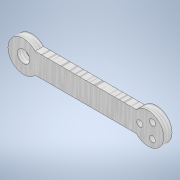
# Autodesk Inventor part: 駆動軸抑え
Saved by Autodesk Inventor 2020.2 (Build 242310000, 310)
## iProperties
Created: 2020-03-15
Part Number: 駆動軸抑え
Material: アルミニウム 7075
Document SubType Name: Modeling
Designer: aoyam
Density: 2.81 g/cm^3
Appearance: サテン - ブラシ仕上げ 重厚
Author: aoyam
Autodesk Inventor part; units mm, degrees
ref_plane "YZ Plane" through (0, 0, 0) normal (1, 0, 0) x (0, 1, 0)
ref_plane "XZ Plane" through (0, 0, 0) normal (0, 1, 0) x (-1, 0, 0)
ref_plane "XY Plane" through (0, 0, 0) normal (0, 0, 1) x (1, 0, 0)
sketch "スケッチ1" plane through (0, 0, 0) normal (0, 0, 1) x (1, 0, 0)
  arc A0 (2.3922, 20.2558) -> (2.3331, 19.9425) centre (4.2654, 19.7401) ccw
  arc A1 (2.759, 21.2362) -> (2.3922, 20.2558) centre (7.5685, 18.8782) ccw
  arc A2 (3.8916, 23.0137) -> (2.759, 21.2362) centre (11.1286, 17.1527) ccw
  arc A3 (-0.0572, 19.9425) -> (-0.1163, 20.2558) centre (-1.9895, 19.7401) ccw
  arc A4 (-0.1163, 20.2558) -> (-0.4831, 21.2362) centre (-5.2926, 18.8782) ccw
  arc A5 (-0.4831, 21.2362) -> (-1.6157, 23.0137) centre (-8.8527, 17.1527) ccw
  arc A6 (2.2508, 18.6513) -> (0.0251, 18.6513) centre (1.1379, 1.1867) ccw
  arc A7 (-1.6157, 23.0137) -> (-2.9881, 22.7963) centre (1.1379, 1.1867) ccw
  line L0 (2.2508, 18.6513) -> (2.3331, 19.9425)
  line L1 (0.0251, 18.6513) -> (-0.0572, 19.9425)
  line L2 (-5.3173, 17.4526) -> (-5.7946, 18.6552)
  arc A8 (-5.7946, 18.6552) -> (-5.9476, 18.9349) centre (-7.5698, 17.8656) ccw
  arc A9 (-5.9476, 18.9349) -> (-6.5994, 19.754) centre (-10.4448, 16.0252) ccw
  arc A10 (-6.5994, 19.754) -> (-8.2258, 21.0945) centre (-13.2975, 13.284) ccw
  arc A11 (-8.2258, 21.0945) -> (-9.4639, 20.4637) centre (1.1379, 1.1867) ccw
  arc A12 (-3.2005, 18.1404) -> (-5.3173, 17.4526) centre (1.1379, 1.1867) ccw
  line L3 (-3.2005, 18.1404) -> (-3.5213, 19.3939)
  arc A13 (-3.5619, 19.71) -> (-3.5213, 19.3939) centre (-1.621, 19.7985) ccw
  arc A14 (-3.516, 20.7559) -> (-3.5619, 19.71) centre (1.7868, 19.9995) ccw
  arc A15 (-2.9881, 22.7963) -> (-3.516, 20.7559) centre (5.7058, 19.4586) ccw
  line L4 (-10.0278, 14.6617) -> (-10.8533, 15.658)
  arc A16 (-10.8533, 15.658) -> (-11.0853, 15.8767) centre (-12.2977, 14.3585) ccw
  arc A17 (-11.0853, 15.8767) -> (-11.9583, 16.4543) centre (-14.4633, 11.7197) ccw
  arc A18 (-11.9583, 16.4543) -> (-13.9194, 17.2266) centre (-16.3293, 8.2311) ccw
  arc A19 (-13.9194, 17.2266) -> (-14.9019, 16.244) centre (1.1379, 1.1867) ccw
  arc A20 (-8.2272, 15.97) -> (-10.0278, 14.6617) centre (1.1379, 1.1867) ccw
  line L5 (-8.2272, 15.97) -> (-8.9196, 17.063)
  arc A21 (-9.0559, 17.3511) -> (-8.9196, 17.063) centre (-7.2373, 18.035) ccw
  arc A22 (-9.3354, 18.3599) -> (-9.0559, 17.3511) centre (-4.0584, 19.2792) ccw
  arc A23 (-9.4639, 20.4637) -> (-9.3354, 18.3599) centre (-0.164, 19.9759) ccw
  line L6 (-13.6453, 10.5518) -> (-14.7383, 11.2442)
  arc A24 (-14.7383, 11.2442) -> (-15.0265, 11.3805) centre (-15.7104, 9.562) ccw
  arc A25 (-15.0265, 11.3805) -> (-16.0353, 11.6601) centre (-16.9545, 6.3831) ccw
  arc A26 (-16.0353, 11.6601) -> (-18.139, 11.7886) centre (-17.6512, 2.4887) ccw
  arc A27 (-18.139, 11.7886) -> (-18.7698, 10.5505) centre (1.1379, 1.1867) ccw
  arc A28 (-12.3371, 12.3525) -> (-13.6453, 10.5518) centre (1.1379, 1.1867) ccw
  line L7 (-12.3371, 12.3525) -> (-13.3333, 13.178)
  arc A29 (-13.552, 13.4099) -> (-13.3333, 13.178) centre (-12.0338, 14.6223) ccw
  arc A30 (-14.1296, 14.283) -> (-13.552, 13.4099) centre (-9.395, 16.7879) ccw
  arc A31 (-14.9019, 16.244) -> (-14.1296, 14.283) centre (-5.9065, 18.6539) ccw
  line L8 (-15.8158, 5.5252) -> (-17.0692, 5.8459)
  arc A32 (-17.0692, 5.8459) -> (-17.3854, 5.8865) centre (-17.4739, 3.9456) ccw
  arc A33 (-17.3854, 5.8865) -> (-18.4312, 5.8407) centre (-17.6748, 0.5379) ccw
  arc A34 (-18.4312, 5.8407) -> (-20.4717, 5.3128) centre (-17.1339, -3.3812) ccw
  arc A35 (-20.4717, 5.3128) -> (-20.6891, 3.9404) centre (1.1379, 1.1867) ccw
  arc A36 (-15.128, 7.642) -> (-15.8158, 5.5252) centre (1.1379, 1.1867) ccw
  line L9 (-15.128, 7.642) -> (-16.3306, 8.1192)
  arc A37 (-16.6102, 8.2722) -> (-16.3306, 8.1192) centre (-15.541, 9.8944) ccw
  arc A38 (-17.4293, 8.924) -> (-16.6102, 8.2722) centre (-13.7005, 12.7695) ccw
  arc A39 (-18.7698, 10.5505) -> (-17.4293, 8.924) centre (-10.9594, 15.6222) ccw
  line L10 (-16.3266, 0.0739) -> (-17.6179, -0.0084)
  arc A40 (-17.6179, -0.0084) -> (-17.9311, -0.0675) centre (-17.4155, -1.9407) ccw
  arc A41 (-17.9311, -0.0675) -> (-18.9116, -0.4343) centre (-16.5535, -5.2438) ccw
  arc A42 (-18.9116, -0.4343) -> (-20.6891, -1.5669) centre (-14.8281, -8.8039) ccw
  arc A43 (-20.6891, -1.5669) -> (-20.4717, -2.9393) centre (1.1379, 1.1867) ccw
  arc A44 (-16.3266, 2.2996) -> (-16.3266, 0.0739) centre (1.1379, 1.1867) ccw
  line L11 (-16.3266, 2.2996) -> (-17.6179, 2.3819)
  arc A45 (-17.9311, 2.441) -> (-17.6179, 2.3819) centre (-17.4155, 4.3142) ccw
  arc A46 (-18.9116, 2.8078) -> (-17.9311, 2.441) centre (-16.5535, 7.6173) ccw
  arc A47 (-20.6891, 3.9404) -> (-18.9116, 2.8078) centre (-14.8281, 11.1774) ccw
  line L12 (-15.128, -5.2685) -> (-16.3306, -5.7458)
  arc A48 (-16.3306, -5.7458) -> (-16.6102, -5.8988) centre (-15.541, -7.521) ccw
  arc A49 (-16.6102, -5.8988) -> (-17.4293, -6.5506) centre (-13.7005, -10.396) ccw
  arc A50 (-17.4293, -6.5506) -> (-18.7698, -8.177) centre (-10.9594, -13.2487) ccw
  arc A51 (-18.7698, -8.177) -> (-18.139, -9.4151) centre (1.1379, 1.1867) ccw
  arc A52 (-15.8158, -3.1517) -> (-15.128, -5.2685) centre (1.1379, 1.1867) ccw
  line L13 (-15.8158, -3.1517) -> (-17.0692, -3.4725)
  arc A53 (-17.3854, -3.5131) -> (-17.0692, -3.4725) centre (-17.4739, -1.5722) ccw
  arc A54 (-18.4312, -3.4672) -> (-17.3854, -3.5131) centre (-17.6748, 1.8356) ccw
  arc A55 (-20.4717, -2.9393) -> (-18.4312, -3.4672) centre (-17.1339, 5.7546) ccw
  line L14 (-12.3371, -9.979) -> (-13.3333, -10.8046)
  arc A56 (-13.3333, -10.8046) -> (-13.552, -11.0365) centre (-12.0338, -12.2489) ccw
  arc A57 (-13.552, -11.0365) -> (-14.1296, -11.9095) centre (-9.395, -14.4145) ccw
  arc A58 (-14.1296, -11.9095) -> (-14.9019, -13.8706) centre (-5.9065, -16.2805) ccw
  arc A59 (-14.9019, -13.8706) -> (-13.9194, -14.8531) centre (1.1379, 1.1867) ccw
  arc A60 (-13.6453, -8.1784) -> (-12.3371, -9.979) centre (1.1379, 1.1867) ccw
  line L15 (-13.6453, -8.1784) -> (-14.7383, -8.8708)
  arc A61 (-15.0265, -9.0071) -> (-14.7383, -8.8708) centre (-15.7104, -7.1885) ccw
  arc A62 (-16.0353, -9.2866) -> (-15.0265, -9.0071) centre (-16.9545, -4.0097) ccw
  arc A63 (-18.139, -9.4151) -> (-16.0353, -9.2866) centre (-17.6512, -0.1153) ccw
  line L16 (-8.2272, -13.5965) -> (-8.9196, -14.6895)
  arc A64 (-8.9196, -14.6895) -> (-9.0559, -14.9777) centre (-7.2373, -15.6616) ccw
  arc A65 (-9.0559, -14.9777) -> (-9.3354, -15.9865) centre (-4.0584, -16.9058) ccw
  arc A66 (-9.3354, -15.9865) -> (-9.4639, -18.0902) centre (-0.164, -17.6024) ccw
  arc A67 (-9.4639, -18.0902) -> (-8.2258, -18.7211) centre (1.1379, 1.1867) ccw
  arc A68 (-10.0278, -12.2883) -> (-8.2272, -13.5965) centre (1.1379, 1.1867) ccw
  line L17 (-10.0278, -12.2883) -> (-10.8533, -13.2846)
  arc A69 (-11.0853, -13.5032) -> (-10.8533, -13.2846) centre (-12.2977, -11.985) ccw
  arc A70 (-11.9583, -14.0808) -> (-11.0853, -13.5032) centre (-14.4633, -9.3462) ccw
  arc A71 (-13.9194, -14.8531) -> (-11.9583, -14.0808) centre (-16.3293, -5.8577) ccw
  line L18 (-3.2005, -15.767) -> (-3.5213, -17.0204)
  arc A72 (-3.5213, -17.0204) -> (-3.5619, -17.3366) centre (-1.621, -17.4251) ccw
  arc A73 (-3.5619, -17.3366) -> (-3.516, -18.3824) centre (1.7868, -17.626) ccw
  arc A74 (-3.516, -18.3824) -> (-2.9881, -20.4229) centre (5.7058, -17.0851) ccw
  arc A75 (-2.9881, -20.4229) -> (-1.6157, -20.6403) centre (1.1379, 1.1867) ccw
  arc A76 (-5.3173, -15.0792) -> (-3.2005, -15.767) centre (1.1379, 1.1867) ccw
  line L19 (-5.3173, -15.0792) -> (-5.7946, -16.2818)
  arc A77 (-5.9476, -16.5614) -> (-5.7946, -16.2818) centre (-7.5698, -15.4922) ccw
  arc A78 (-6.5994, -17.3806) -> (-5.9476, -16.5614) centre (-10.4448, -13.6517) ccw
  arc A79 (-8.2258, -18.7211) -> (-6.5994, -17.3806) centre (-13.2975, -10.9106) ccw
  line L20 (2.2508, -16.2779) -> (2.3331, -17.5691)
  arc A80 (2.3331, -17.5691) -> (2.3922, -17.8823) centre (4.2654, -17.3667) ccw
  arc A81 (2.3922, -17.8823) -> (2.759, -18.8628) centre (7.5685, -16.5048) ccw
  arc A82 (2.759, -18.8628) -> (3.8916, -20.6403) centre (11.1286, -14.7793) ccw
  arc A83 (3.8916, -20.6403) -> (5.264, -20.4229) centre (1.1379, 1.1867) ccw
  arc A84 (0.0251, -16.2779) -> (2.2508, -16.2779) centre (1.1379, 1.1867) ccw
  line L21 (0.0251, -16.2779) -> (-0.0572, -17.5691)
  arc A85 (-0.1163, -17.8823) -> (-0.0572, -17.5691) centre (-1.9895, -17.3667) ccw
  arc A86 (-0.4831, -18.8628) -> (-0.1163, -17.8823) centre (-5.2926, -16.5048) ccw
  arc A87 (-1.6157, -20.6403) -> (-0.4831, -18.8628) centre (-8.8527, -14.7793) ccw
  line L22 (7.5932, -15.0792) -> (8.0705, -16.2818)
  arc A88 (8.0705, -16.2818) -> (8.2235, -16.5614) centre (9.8457, -15.4922) ccw
  arc A89 (8.2235, -16.5614) -> (8.8753, -17.3806) centre (12.7207, -13.6517) ccw
  arc A90 (8.8753, -17.3806) -> (10.5017, -18.7211) centre (15.5734, -10.9106) ccw
  arc A91 (10.5017, -18.7211) -> (11.7398, -18.0902) centre (1.1379, 1.1867) ccw
  arc A92 (5.4764, -15.767) -> (7.5932, -15.0792) centre (1.1379, 1.1867) ccw
  line L23 (5.4764, -15.767) -> (5.7971, -17.0204)
  arc A93 (5.8377, -17.3366) -> (5.7971, -17.0204) centre (3.8969, -17.4251) ccw
  arc A94 (5.7919, -18.3824) -> (5.8377, -17.3366) centre (0.4891, -17.626) ccw
  arc A95 (5.264, -20.4229) -> (5.7919, -18.3824) centre (-3.43, -17.0851) ccw
  line L24 (12.3037, -12.2883) -> (13.1292, -13.2846)
  arc A96 (13.1292, -13.2846) -> (13.3611, -13.5032) centre (14.5735, -11.985) ccw
  arc A97 (13.3611, -13.5032) -> (14.2342, -14.0808) centre (16.7391, -9.3462) ccw
  arc A98 (14.2342, -14.0808) -> (16.1953, -14.8531) centre (18.6051, -5.8577) ccw
  arc A99 (16.1953, -14.8531) -> (17.1778, -13.8706) centre (1.1379, 1.1867) ccw
  arc A100 (10.503, -13.5965) -> (12.3037, -12.2883) centre (1.1379, 1.1867) ccw
  line L25 (10.503, -13.5965) -> (11.1954, -14.6895)
  arc A101 (11.3317, -14.9777) -> (11.1954, -14.6895) centre (9.5132, -15.6616) ccw
  arc A102 (11.6113, -15.9865) -> (11.3317, -14.9777) centre (6.3343, -16.9058) ccw
  arc A103 (11.7398, -18.0902) -> (11.6113, -15.9865) centre (2.4399, -17.6024) ccw
  line L26 (15.9212, -8.1784) -> (17.0142, -8.8708)
  arc A104 (17.0142, -8.8708) -> (17.3023, -9.0071) centre (17.9862, -7.1885) ccw
  arc A105 (17.3023, -9.0071) -> (18.3111, -9.2866) centre (19.2304, -4.0097) ccw
  arc A106 (18.3111, -9.2866) -> (20.4149, -9.4151) centre (19.9271, -0.1153) ccw
  arc A107 (20.4149, -9.4151) -> (21.0457, -8.177) centre (1.1379, 1.1867) ccw
  arc A108 (14.6129, -9.979) -> (15.9212, -8.1784) centre (1.1379, 1.1867) ccw
  line L27 (14.6129, -9.979) -> (15.6092, -10.8046)
  arc A109 (15.8279, -11.0365) -> (15.6092, -10.8046) centre (14.3097, -12.2489) ccw
  arc A110 (16.4055, -11.9095) -> (15.8279, -11.0365) centre (11.6709, -14.4145) ccw
  arc A111 (17.1778, -13.8706) -> (16.4055, -11.9095) centre (8.1824, -16.2805) ccw
  line L28 (18.0916, -3.1517) -> (19.3451, -3.4725)
  arc A112 (19.3451, -3.4725) -> (19.6613, -3.5131) centre (19.7497, -1.5722) ccw
  arc A113 (19.6613, -3.5131) -> (20.7071, -3.4672) centre (19.9507, 1.8356) ccw
  arc A114 (20.7071, -3.4672) -> (22.7476, -2.9393) centre (19.4098, 5.7546) ccw
  arc A115 (22.7476, -2.9393) -> (22.9649, -1.5669) centre (1.1379, 1.1867) ccw
  arc A116 (17.4038, -5.2685) -> (18.0916, -3.1517) centre (1.1379, 1.1867) ccw
  line L29 (17.4038, -5.2685) -> (18.6065, -5.7458)
  arc A117 (18.8861, -5.8988) -> (18.6065, -5.7458) centre (17.8168, -7.521) ccw
  arc A118 (19.7052, -6.5506) -> (18.8861, -5.8988) centre (15.9764, -10.396) ccw
  arc A119 (21.0457, -8.177) -> (19.7052, -6.5506) centre (13.2352, -13.2487) ccw
  line L30 (18.6025, 2.2996) -> (19.8937, 2.3819)
  arc A120 (19.8937, 2.3819) -> (20.207, 2.441) centre (19.6914, 4.3142) ccw
  arc A121 (20.207, 2.441) -> (21.1874, 2.8078) centre (18.8294, 7.6173) ccw
  arc A122 (21.1874, 2.8078) -> (22.9649, 3.9404) centre (17.104, 11.1774) ccw
  arc A123 (22.9649, 3.9404) -> (22.7476, 5.3128) centre (1.1379, 1.1867) ccw
  arc A124 (18.6025, 0.0739) -> (18.6025, 2.2996) centre (1.1379, 1.1867) ccw
  line L31 (18.6025, 0.0739) -> (19.8937, -0.0084)
  arc A125 (20.207, -0.0675) -> (19.8937, -0.0084) centre (19.6914, -1.9407) ccw
  arc A126 (21.1874, -0.4343) -> (20.207, -0.0675) centre (18.8294, -5.2438) ccw
  arc A127 (22.9649, -1.5669) -> (21.1874, -0.4343) centre (17.104, -8.8039) ccw
  line L32 (17.4038, 7.642) -> (18.6065, 8.1192)
  arc A128 (18.6065, 8.1192) -> (18.8861, 8.2722) centre (17.8168, 9.8944) ccw
  arc A129 (18.8861, 8.2722) -> (19.7052, 8.924) centre (15.9764, 12.7695) ccw
  arc A130 (19.7052, 8.924) -> (21.0457, 10.5505) centre (13.2352, 15.6222) ccw
  arc A131 (21.0457, 10.5505) -> (20.4149, 11.7886) centre (1.1379, 1.1867) ccw
  arc A132 (18.0916, 5.5252) -> (17.4038, 7.642) centre (1.1379, 1.1867) ccw
  line L33 (18.0916, 5.5252) -> (19.3451, 5.8459)
  arc A133 (19.6613, 5.8865) -> (19.3451, 5.8459) centre (19.7497, 3.9456) ccw
  arc A134 (20.7071, 5.8407) -> (19.6613, 5.8865) centre (19.9507, 0.5379) ccw
  arc A135 (22.7476, 5.3128) -> (20.7071, 5.8407) centre (19.4098, -3.3812) ccw
  line L34 (14.6129, 12.3525) -> (15.6092, 13.178)
  arc A136 (15.6092, 13.178) -> (15.8279, 13.4099) centre (14.3097, 14.6223) ccw
  arc A137 (15.8279, 13.4099) -> (16.4055, 14.283) centre (11.6709, 16.7879) ccw
  arc A138 (16.4055, 14.283) -> (17.1778, 16.244) centre (8.1824, 18.6539) ccw
  arc A139 (17.1778, 16.244) -> (16.1953, 17.2266) centre (1.1379, 1.1867) ccw
  arc A140 (15.9212, 10.5518) -> (14.6129, 12.3525) centre (1.1379, 1.1867) ccw
  line L35 (15.9212, 10.5518) -> (17.0142, 11.2442)
  arc A141 (17.3023, 11.3805) -> (17.0142, 11.2442) centre (17.9862, 9.562) ccw
  arc A142 (18.3111, 11.6601) -> (17.3023, 11.3805) centre (19.2304, 6.3831) ccw
  arc A143 (20.4149, 11.7886) -> (18.3111, 11.6601) centre (19.9271, 2.4887) ccw
  line L36 (10.503, 15.97) -> (11.1954, 17.063)
  arc A144 (11.1954, 17.063) -> (11.3317, 17.3511) centre (9.5132, 18.035) ccw
  arc A145 (11.3317, 17.3511) -> (11.6113, 18.3599) centre (6.3343, 19.2792) ccw
  arc A146 (11.6113, 18.3599) -> (11.7398, 20.4637) centre (2.4399, 19.9759) ccw
  arc A147 (11.7398, 20.4637) -> (10.5017, 21.0945) centre (1.1379, 1.1867) ccw
  arc A148 (12.3037, 14.6617) -> (10.503, 15.97) centre (1.1379, 1.1867) ccw
  line L37 (12.3037, 14.6617) -> (13.1292, 15.658)
  arc A149 (13.3611, 15.8767) -> (13.1292, 15.658) centre (14.5735, 14.3585) ccw
  arc A150 (14.2342, 16.4543) -> (13.3611, 15.8767) centre (16.7391, 11.7197) ccw
  arc A151 (16.1953, 17.2266) -> (14.2342, 16.4543) centre (18.6051, 8.2311) ccw
  line L38 (5.4764, 18.1404) -> (5.7971, 19.3939)
  arc A152 (5.7971, 19.3939) -> (5.8377, 19.71) centre (3.8969, 19.7985) ccw
  arc A153 (5.8377, 19.71) -> (5.7919, 20.7559) centre (0.4891, 19.9995) ccw
  arc A154 (5.7919, 20.7559) -> (5.264, 22.7963) centre (-3.43, 19.4586) ccw
  arc A155 (5.264, 22.7963) -> (3.8916, 23.0137) centre (1.1379, 1.1867) ccw
  arc A156 (7.5932, 17.4526) -> (5.4764, 18.1404) centre (1.1379, 1.1867) ccw
  line L39 (7.5932, 17.4526) -> (8.0705, 18.6552)
  arc A157 (8.2235, 18.9349) -> (8.0705, 18.6552) centre (9.8457, 17.8656) ccw
  arc A158 (8.8753, 19.754) -> (8.2235, 18.9349) centre (12.7207, 16.0252) ccw
  arc A159 (10.5017, 21.0945) -> (8.8753, 19.754) centre (15.5734, 13.284) ccw
  circle A160 centre (1.1379, 1.1867) radius 3.025
  line L40 (1.1379, 1.1867) -> (61.1379, 1.1867)
  line L41 (66.1379, -3.8133) -> (-5.7946, -3.8133)
  line L42 (-5.7946, -3.8133) -> (-5.7946, 6.1867)
  line L43 (-5.7946, 6.1867) -> (66.1379, 6.1867)
  line L44 (66.1379, 6.1867) -> (66.1379, -3.8133)
  circle A161 centre (61.1379, 1.1867) radius 7.5
  circle A162 centre (1.1379, 1.1867) radius 7.5
  circle A163 centre (57.1379, 1.1867) radius 1.5
  circle A164 centre (63.1379, -2.2774) radius 1.5
  circle A165 centre (63.1379, 4.6508) radius 1.5
  line L45 (63.1379, -2.2774) -> (63.1379, 4.6508)
  point P0 (0, 0)
  point P1 (-10.0278, -12.2883)
  point P2 (-8.2272, -13.5965)
  point P3 (-8.9196, -14.6895)
  point P4 (-9.0559, -14.9777)
  point P5 (-9.3354, -15.9865)
  point P6 (-9.4639, -18.0902)
  point P7 (-8.2258, -18.7211)
  point P8 (-5.9476, -16.5614)
  point P9 (-5.7946, -16.2818)
  point P10 (-5.3173, -15.0792)
  point P11 (-3.2005, -15.767)
  point P12 (-3.5213, -17.0204)
  point P13 (-3.5619, -17.3366)
  point P14 (-3.516, -18.3824)
  point P15 (-2.9881, -20.4229)
  point P16 (-1.6157, -20.6403)
  point P17 (-0.4831, -18.8628)
  point P18 (-0.1163, -17.8823)
  point P19 (-0.0572, -17.5691)
  point P20 (0.0251, -16.2779)
  point P21 (2.2508, -16.2779)
  point P22 (2.3331, -17.5691)
  point P23 (2.3922, -17.8823)
  point P24 (2.759, -18.8628)
  point P25 (3.8916, -20.6403)
  point P26 (5.264, -20.4229)
  point P27 (5.7919, -18.3824)
  point P28 (5.8377, -17.3366)
  point P29 (5.4764, -15.767)
  point P30 (7.5932, -15.0792)
  point P31 (8.2235, -16.5614)
  point P32 (8.8753, -17.3806)
  point P33 (10.5017, -18.7211)
  point P34 (11.7398, -18.0902)
  point P35 (11.6113, -15.9865)
  point P36 (11.3317, -14.9777)
  point P37 (10.503, -13.5965)
  point P38 (13.3611, -13.5032)
  point P39 (14.2342, -14.0808)
  point P40 (16.1953, -14.8531)
  point P41 (17.1778, -13.8706)
  point P42 (16.4055, -11.9095)
  point P43 (15.8279, -11.0365)
  point P44 (14.6129, -9.979)
  point P45 (17.3023, -9.0071)
  point P46 (18.3111, -9.2866)
  point P47 (20.4149, -9.4151)
  point P48 (21.0457, -8.177)
  point P49 (19.7052, -6.5506)
  point P50 (18.8861, -5.8988)
  point P51 (17.4038, -5.2685)
  point P52 (19.6613, -3.5131)
  point P53 (20.7071, -3.4672)
  point P54 (22.7476, -2.9393)
  point P55 (22.9649, -1.5669)
  point P56 (21.1874, -0.4343)
  point P57 (20.207, -0.0675)
  point P58 (18.6025, 0.0739)
  point P59 (20.207, 2.441)
  point P60 (21.1874, 2.8078)
  point P61 (22.9649, 3.9404)
  point P62 (20.7071, 5.8407)
  point P63 (19.6613, 5.8865)
  point P64 (19.3451, 5.8459)
  point P65 (17.4038, 7.642)
  point P66 (18.6065, 8.1192)
  point P67 (18.8861, 8.2722)
  point P68 (19.7052, 8.924)
  point P69 (21.0457, 10.5505)
  point P70 (20.4149, 11.7886)
  point P71 (18.3111, 11.6601)
  point P72 (17.3023, 11.3805)
  point P73 (15.8279, 13.4099)
  point P74 (16.4055, 14.283)
  point P75 (17.1778, 16.244)
  point P76 (16.1953, 17.2266)
  point P77 (14.2342, 16.4543)
  point P78 (13.3611, 15.8767)
  point P79 (12.3037, 14.6617)
  point P80 (10.503, 15.97)
  point P81 (11.1954, 17.063)
  point P82 (11.3317, 17.3511)
  point P83 (11.6113, 18.3599)
  point P84 (11.7398, 20.4637)
  point P85 (10.5017, 21.0945)
  point P86 (8.8753, 19.754)
  point P87 (8.2235, 18.9349)
  point P88 (8.0705, 18.6552)
  point P89 (5.8377, 19.71)
  point P90 (5.7919, 20.7559)
  point P91 (5.264, 22.7963)
  point P92 (3.8916, 23.0137)
  point P93 (2.759, 21.2362)
  point P94 (2.3922, 20.2558)
  point P95 (-0.1163, 20.2558)
  point P96 (-0.4831, 21.2362)
  point P97 (-1.6157, 23.0137)
  point P98 (-2.9881, 22.7963)
  point P99 (-3.516, 20.7559)
  point P100 (-3.5619, 19.71)
  point P101 (-3.5213, 19.3939)
  point P102 (-3.2005, 18.1404)
  point P103 (-5.3173, 17.4526)
  point P104 (-5.7946, 18.6552)
  point P105 (-5.9476, 18.9349)
  point P106 (-6.5994, 19.754)
  point P107 (-8.2258, 21.0945)
  point P108 (-9.4639, 20.4637)
  point P109 (-9.3354, 18.3599)
  point P110 (-9.0559, 17.3511)
  point P111 (-8.9196, 17.063)
  point P112 (-10.0278, 14.6617)
  point P113 (-10.8533, 15.658)
  point P114 (-11.0853, 15.8767)
  point P115 (-11.9583, 16.4543)
  point P116 (-13.9194, 17.2266)
  point P117 (-14.9019, 16.244)
  point P118 (-14.1296, 14.283)
  point P119 (-13.552, 13.4099)
  point P120 (-14.7383, 11.2442)
  point P121 (-15.0265, 11.3805)
  point P122 (-16.0353, 11.6601)
  point P123 (-18.139, 11.7886)
  point P124 (-18.7698, 10.5505)
  point P125 (-17.4293, 8.924)
  point P126 (-16.6102, 8.2722)
  point P127 (-15.8158, 5.5252)
  point P128 (-17.0692, 5.8459)
  point P129 (-17.3854, 5.8865)
  point P130 (-18.4312, 5.8407)
  point P131 (-20.4717, 5.3128)
  point P132 (-20.6891, 3.9404)
  point P133 (-18.9116, 2.8078)
  point P134 (-17.9311, 2.441)
  point P135 (-17.6179, -0.0084)
  point P136 (-17.9311, -0.0675)
  point P137 (-18.9116, -0.4343)
  point P138 (-20.6891, -1.5669)
  point P139 (-18.4312, -3.4672)
  point P140 (-17.3854, -3.5131)
  point P141 (-15.8158, -3.1517)
  point P142 (-15.128, -5.2685)
  point P143 (-16.3306, -5.7458)
  point P144 (-16.6102, -5.8988)
  point P145 (-17.4293, -6.5506)
  point P146 (-18.7698, -8.177)
  point P147 (-18.139, -9.4151)
  point P148 (-16.0353, -9.2866)
  point P149 (-15.0265, -9.0071)
  point P150 (-14.7383, -8.8708)
  point P151 (-13.6453, -8.1784)
  point P152 (-12.3371, -9.979)
  point P153 (-13.3333, -10.8046)
  point P154 (-13.552, -11.0365)
  point P155 (-14.1296, -11.9095)
  point P156 (-14.9019, -13.8706)
  point P157 (-13.9194, -14.8531)
  point P158 (-11.9583, -14.0808)
  point P159 (-11.0853, -13.5032)
  point P160 (-10.8533, -13.2846)
  point P161 (17.9084, -3.8133)
  point P162 (17.9084, 6.1867)
  point P163 (55.5478, -3.8133)
  point P164 (55.5478, 6.1867)
  point P165 (6.7281, -3.8133)
  point P166 (6.7281, 6.1867)
  dimension "d2" = 360
  dimension "d4" = 6.05
  dimension "d7" = 60
  dimension "d9" = 15
  dimension "d10" = 15
  dimension "d11" = 3
  dimension "d12" = 4
  dimension "d15" = 360
  constraints: 320 point on circle, 166 centre point, 92 end point, 5 coincident, 3 horizontal, 2 parallel, 1 perpendicular, 1 point on line, 1 vertical, 767 other
  measures "d4" diameter of A160
  measures "d7" distance of L40.start L40.end
  measures "d9" diameter of A161
  measures "d10" diameter of A162
  measures "d11" diameter of A163
  measures "d12" distance of A161.centre A163.centre
extrude "押し出し1" add sketch "スケッチ1" along normal blind 4 contours L43 A161 L40 A124 L30 A120 A121 A122 A123 A135 A134 A133 L33 A132 | A132 L33 A133 A134 A135 A123 A122 A121 A120 L30 A124 L40 A162 L43 | A162 L41 L42 L43 | L43 A162 | A161 L41 L44 L43 | L43 L44 L41 A161 | L40 A124 L31 A125 A126 A127 A115 A114 A113 A112 L28 A116 L41 A162 | A161 L41 A116 L28 A112 A113 A114 A115 A127 A126 A125 L31 A124 L40 | L42 A162 | A162 L41
